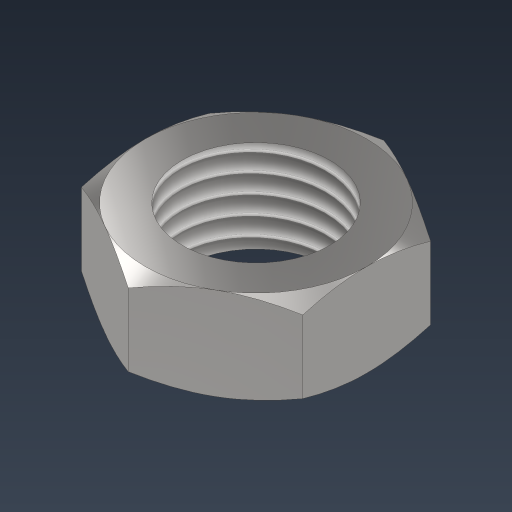
# Autodesk Inventor part: csavar
Saved by Autodesk Inventor 2024.3 (Build 283343000, 343)
## iProperties
Created: 2025-10-06
Part Number: csavar
Material: Steel, Alloy
Document SubType Name: Modeling
Designer: Agi
Density: 7.73 g/cm^3
Appearance: Semi-Polished
Author: Agi
Autodesk Inventor part; units mm, degrees
ref_plane "YZ Plane" through (0, 0, 0) normal (1, 0, 0) x (0, 1, 0)
ref_plane "XZ Plane" through (0, 0, 0) normal (0, 1, 0) x (-1, 0, 0)
ref_plane "XY Plane" through (0, 0, 0) normal (0, 0, 1) x (1, 0, 0)
sketch "Sketch1" plane through (0, 0, 0) normal (0, 1, 0) x (-1, 0, 0)
  line L0 (12, -6.9282) -> (0, -13.8564)
  line L1 (0, -13.8564) -> (-12, -6.9282)
  line L2 (-12, -6.9282) -> (-12, 6.9282)
  line L3 (-12, 6.9282) -> (0, 13.8564)
  line L4 (0, 13.8564) -> (12, 6.9282)
  line L5 (12, 6.9282) -> (12, -6.9282)
  point P0 (0, 0)
  point P1 (0, 0)
  point P2 (-12, 0)
  point P3 (12, 0)
  dimension "d0" = 24
  constraints: 12 end point, 2 midpoint, 1 coincident, 1 vertical, 13 other
  measures "d0" distance of point (-12, 0) point (12, 0)
extrude "Extrusion1" add sketch "Sketch1" along normal blind 10
sketch "Sketch2" plane through (0, 10, 0) normal (0, 1, 0) x (1, 0, 0)
  circle A0 centre (0, 0) radius 12
  constraints: 1 centre point, 1 coincident, 1 other
extrude "Extrusion2" cut sketch "Sketch2" against normal blind 10 draft 60 keep common part
sketch "Sketch4" plane through (0, 0, 0) normal (0, -1, 0) x (1, 0, 0)
  circle A0 centre (0, 0) radius 12
  constraints: 1 centre point, 1 coincident
extrude "Extrusion4" cut sketch "Sketch4" against normal blind 60 draft 60 keep common part
sketch "Sketch5" plane through (0, 10, 0) normal (0, 1, 0) x (1, 0, 0)
  point P0 (0, 0)
  point P1 (0, 0)
  constraints: 1 coincident
hole "Hole1" at (0, 10, 0) direction (0, -1, 0) diameter 16 end through all
thread "Thread2" size "M16x2" class "6H" standard "ANSI Metric M Profile" length 38
body "Solid1"
